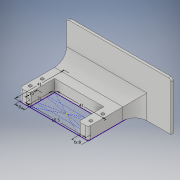
# Autodesk Inventor part: servoholder
Saved by Autodesk Inventor 2019 (Build 230136000, 136)
## iProperties
Created: 2019-02-25
Part Number: servoholder
Material: Generic
Document SubType Name: Modeling
Designer: erwin
Density: 1 g/cm^3
Appearance: Default
Author: erwin
Autodesk Inventor part; units mm, degrees
ref_plane "YZ Plane" through (0, 0, 0) normal (1, 0, 0) x (0, 1, 0)
ref_plane "XZ Plane" through (0, 0, 0) normal (0, 1, 0) x (-1, 0, 0)
ref_plane "XY Plane" through (0, 0, 0) normal (0, 0, 1) x (1, 0, 0)
sketch "Sketch1" plane through (0, 0, 0) normal (0, 1, 0) x (-1, 0, 0)
  line L0 (-20.5, 10.5) -> (20.5, 10.5)
  line L1 (20.5, 10.5) -> (20.5, -10.5)
  line L2 (20.5, -10.5) -> (-20.5, -10.5)
  line L3 (-20.5, -10.5) -> (-20.5, 10.5)
  line L4 (-20.5, 10.5) -> (20.5, -10.5) construction
  line L5 (20.5, 10.5) -> (-20.5, -10.5) construction
  line L6 (20.5, 10.5) -> (28.5, 10.5)
  line L7 (28.5, 10.5) -> (28.5, -30.5)
  line L8 (28.5, -30.5) -> (-28.5, -30.5)
  line L9 (-28.5, -30.5) -> (-28.5, 10.5)
  line L10 (-28.5, 10.5) -> (-20.5, 10.5)
  line L11 (-25.25, -5) -> (25.25, -5) construction
  line L12 (25.25, -5) -> (25.25, 5) construction
  line L13 (25.25, 5) -> (-25.25, 5) construction
  line L14 (-25.25, 5) -> (-25.25, -5) construction
  line L15 (-25.25, -5) -> (25.25, 5) construction
  line L16 (25.25, -5) -> (-25.25, 5) construction
  point P0 (0, 0)
  dimension "d0" = 41
  dimension "d1" = 21
  dimension "d2" = 8
  dimension "d3" = 41
  dimension "d4" = 8
  dimension "d5" = 50.5
  dimension "d6" = 10
  constraints: 34 end point, 6 perpendicular, 4 coincident, 4 midpoint, 4 parallel, 3 horizontal, 1 point on line
  measures "d0" distance of L1.end L2.end
  measures "d1" distance of L0.end L1.end
  measures "d2" distance of L0.end L6.end
  measures "d3" distance of L6.end L7.end
  measures "d4" distance of L9.end L0.start
  measures "d5" distance of L13.end L12.end
  measures "d6" distance of L12.end L11.end
extrude "Extrusion1" add sketch "Sketch1" along normal blind 10 contours L3 L2 L1 L6 L7 L8 L9 L10
hole "Hole1" at (-25.25, 0, 5) at (-25.25, 0, -5) at (25.25, 0, 5) at (25.25, 0, -5) direction (0, 1, 0) diameter 2.5 end through all both
sketch "Sketch2" plane through (0, 10, 0) normal (0, 1, 0) x (1, 0, 0)
  line L0 (-28.5, 30.5) -> (-28.5, -10.5) projected
  line L1 (28.5, -10.5) -> (28.5, 30.5) projected
  line L2 (-28.5, 30.5) -> (28.5, 30.5)
  line L3 (28.5, 30.5) -> (28.5, 28.5)
  line L4 (28.5, 28.5) -> (-28.5, 28.5)
  line L5 (-28.5, 28.5) -> (-28.5, 30.5)
  point P0 (0, 0)
  dimension "d16" = 2
  constraints: 8 end point, 2 parallel, 1 horizontal, 1 perpendicular, 1 point on line
  measures "d16" distance of L2.end L3.end
extrude "Extrusion2" add sketch "Sketch2" along normal blind 30
sketch "Sketch3" plane through (28.5, 0, 10.5) normal (1, 0, 0) x (0, 0, -1)
  line L0 (39, 10) -> (39, 40) projected
  line L1 (41.007, 0) -> (39, 0)
  line L2 (39, 0) -> (39, 40)
  line L3 (39, 40) -> (41.007, 40)
  line L4 (41.007, 40) -> (41.007, 0)
  point P0 (10.5, 0)
  constraints: 8 end point, 2 parallel, 1 horizontal, 1 perpendicular
extrude "Extrusion3" add sketch "Sketch3" along normal blind 30
fillet "Fillet2" radius 10 2 edges at (28.5, 5, -28.5) (0, 10, -28.5)
fillet "Fillet2" radius 2 6 edges at (58.5, 40, -29.5035) (-28.5, 40, -29.5) (28.5, 5, 10.5) (20.5, 5, 10.5) (-20.5, 5, 10.5) (-28.5, 5, 10.5)
equation "\"d4\" = d2"
body "Solid1"
